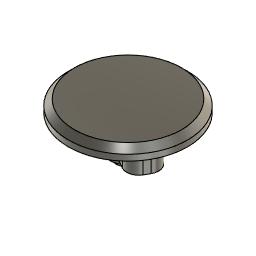
Scale_Hub_Long v2 (Autodesk Fusion 360 archive; units mm, degrees)
design "scaleHUB"
Autodesk Fusion 360 part; units mm, degrees
sketch "Sketch1" plane through (0, 0, 0) normal (0, 0, 1) x (1, 0, 0)
  line L0 (-2, 1.8875) -> (-2, -1.8875)
  line L1 (2, -1.8875) -> (2, 1.8875)
  line L2 (1.0213, 2.5533) -> (-1.0213, -2.5533) construction
  line L3 (-1.0213, 2.5533) -> (1.0213, -2.5533) construction
  arc A0 (2, 1.8875) -> (-2, 1.8875) centre (0, 0) ccw
  arc A1 (-2, -1.8875) -> (2, -1.8875) centre (0, 0) ccw
  circle A2 centre (0, 0) radius 6
  dimension "d1" = 5.5
  dimension "d4" = 12
  constraint coincident A0.centre A1.centre
  constraint parallel L0 L1
  constraint coincident L2 A0.centre
  constraint coincident L3 A0.centre
  constraint coincident L2.start A0
  constraint coincident L3.start A0
  constraint coincident L0.end A0
  constraint coincident L2.end A0
  constraint coincident L3.end A0
  constraint concentric A0 A1
  constraint concentric A0 A2
  measures "d1" diameter of A0
  measures "d4" diameter of A2
extrude "Extrude1" add sketch "Sketch1" along normal blind 7
chamfer "Chamfer1" distance 2 angle 45 1 edges at (-5.594, -2.1697, 0)
sketch "Sketch2" plane through (0, 0, 7) normal (0, 0, 1) x (-1, 0, 0)
  arc A0 (2, 1.8875) -> (-2, 1.8875) centre (0, 0) ccw
  line L0 (2, 1.8875) -> (2, -1.8875)
  arc A1 (-2, -1.8875) -> (2, -1.8875) centre (0, 0) ccw
  line L1 (-2, -1.8875) -> (-2, 1.8875)
  circle A2 centre (0, 0) radius 6
  circle A3 centre (0, 0) radius 7.5
  dimension "d8" = 15
  constraint coincident A0.centre A1.centre
  measures "d8" diameter of A3
extrude "Extrude2" add sketch "Sketch2" along normal blind 6 contours A2 | A3
sketch "Sketch3" plane through (0, 0, 13) normal (0, 0, 1) x (-1, 0, 0)
  arc A0 (2, 1.8875) -> (-2, 1.8875) centre (0, 0) ccw
  line L0 (2, 1.8875) -> (2, -1.8875)
  arc A1 (-2, -1.8875) -> (2, -1.8875) centre (0, 0) ccw
  line L1 (-2, -1.8875) -> (-2, 1.8875)
  circle A2 centre (0, 0) radius 7.5
  line L2 (0, -7.5) -> (0, -17.5) construction
  line L3 (0, -17.5) -> (5, -17.5) construction
  line L4 (5, -17.5) -> (-5, -17.5) construction
  line L5 (-5, -17.5) -> (-5, -5.5902) construction
  line L6 (5, -17.5) -> (5, -5.5902) construction
  line L7 (5, -5.5902) -> (5, -17.5)
  line L8 (-5, -17.5) -> (-5, -5.5902)
  line L9 (-5, -17.5) -> (5, -17.5)
  line L10 (17.6554, 4.4199) -> (7.3412, -1.535)
  line L11 (17.6554, 4.4199) -> (12.6554, 13.0801)
  line L12 (12.6554, 13.0801) -> (2.3412, 7.1252) construction
  line L13 (-12.6554, 13.0801) -> (-2.3412, 7.1252)
  line L14 (-12.6554, 13.0801) -> (-17.6554, 4.4199)
  line L15 (-17.6554, 4.4199) -> (-7.3412, -1.535) construction
  line L16 (-7.3412, -1.535) -> (-17.6554, 4.4199)
  line L17 (2.3412, 7.1252) -> (12.6554, 13.0801)
  dimension "d11" = 10
  dimension "d12" = 5
  dimension "d18" = 360
  constraint coincident A2 L2.start
  constraint vertical L2
  constraint perpendicular L2 L3
  constraint perpendicular L2 L4
  constraint coincident A2 L5.end
  constraint perpendicular L4 L5
  constraint coincident A2 L6.end
  constraint perpendicular L4 L6
  measures "d11" distance of L2.start L2.end
  measures "d12" distance of L2.end L3.end
extrude "Extrude3" add sketch "Sketch3" against normal blind 6 contours A2 L7 L8 L9
fillet "Fillet1" radius 5 2 edges at (5, 17.5, 10) (-5, 17.5, 10)
extrude "Extrude4" add sketch "Sketch3" against normal blind 6 contours A2 L10 L11 L17 | A2 L13 L14 L16 | A2 L7 L8 L9
fillet "Fillet2" radius 4 6 edges at (-5, 17.5, 10) (5, 17.5, 10) (17.6554, -4.4199, 10) (12.6554, -13.0801, 10) (-12.6554, -13.0801, 10) (-17.6554, -4.4199, 10)
sketch "Sketch4" plane through (0, 0, 13) normal (0, 0, 1) x (-1, 0, 0)
  arc A0 (14.1913, 2.4199) -> (15.6554, 7.884) centre (12.1913, 5.884) ccw
  line L0 (15.6554, 7.884) -> (14.6554, 9.616)
  arc A1 (14.6554, 9.616) -> (9.1913, 11.0801) centre (11.1913, 7.616) ccw
  line L1 (9.1913, 11.0801) -> (2.3412, 7.1252)
  arc A2 (2.3412, 7.1252) -> (-2.3412, 7.1252) centre (0, 0) ccw
  line L2 (-2.3412, 7.1252) -> (-9.1913, 11.0801)
  arc A3 (-9.1913, 11.0801) -> (-14.6554, 9.616) centre (-11.1913, 7.616) ccw
  line L3 (-14.6554, 9.616) -> (-15.6554, 7.884)
  arc A4 (-15.6554, 7.884) -> (-14.1913, 2.4199) centre (-12.1913, 5.884) ccw
  line L4 (-14.1913, 2.4199) -> (-7.3412, -1.535)
  arc A5 (-7.3412, -1.535) -> (-5, -5.5902) centre (0, 0) ccw
  line L5 (-5, -5.5902) -> (-5, -13.5)
  arc A6 (-5, -13.5) -> (-1, -17.5) centre (-1, -13.5) ccw
  line L6 (-1, -17.5) -> (1, -17.5)
  arc A7 (1, -17.5) -> (5, -13.5) centre (1, -13.5) ccw
  line L7 (5, -13.5) -> (5, -5.5902)
  arc A8 (5, -5.5902) -> (7.3412, -1.535) centre (0, 0) ccw
  line L8 (7.3412, -1.535) -> (14.1913, 2.4199)
  arc A9 (2, 1.8875) -> (-2, 1.8875) centre (0, 0) ccw
  line L9 (2, 1.8875) -> (2, -1.8875)
  arc A10 (-2, -1.8875) -> (2, -1.8875) centre (0, 0) ccw
  line L10 (-2, -1.8875) -> (-2, 1.8875)
  circle A11 centre (0, 0) radius 20
  dimension "d23" = 40
  constraint concentric A2 A11
  measures "d23" diameter of A11
extrude "Extrude5" add sketch "Sketch4" along normal blind 4 contours A0 L0 A1 L1 A2 L2 A3 L3 A4 L4 A5 L5 A6 L6 A7 L7 A8 L8 | A9 L9 A10 L10 | A11
chamfer "Chamfer2" distance 2 angle 45 1 edges at (18.6465, 7.2323, 17)
sketch "Sketch5" plane through (0, 0, 7) normal (0, 0, -1) x (1, 0, 0)
  arc A0 (-15.6554, 7.884) -> (-14.1913, 2.4199) centre (-12.1913, 5.884) ccw
  line L0 (-14.1913, 2.4199) -> (-7.3412, -1.535)
  arc A1 (-7.3412, -1.535) -> (-5, -5.5902) centre (0, 0) ccw
  line L1 (-5, -5.5902) -> (-5, -13.5)
  arc A2 (-5, -13.5) -> (-1, -17.5) centre (-1, -13.5) ccw
  line L2 (-1, -17.5) -> (1, -17.5)
  arc A3 (1, -17.5) -> (5, -13.5) centre (1, -13.5) ccw
  line L3 (5, -13.5) -> (5, -5.5902)
  arc A4 (5, -5.5902) -> (7.3412, -1.535) centre (0, 0) ccw
  line L4 (7.3412, -1.535) -> (14.1913, 2.4199)
  arc A5 (14.1913, 2.4199) -> (15.6554, 7.884) centre (12.1913, 5.884) ccw
  line L5 (15.6554, 7.884) -> (14.6554, 9.616)
  arc A6 (14.6554, 9.616) -> (9.1913, 11.0801) centre (11.1913, 7.616) ccw
  line L6 (9.1913, 11.0801) -> (2.3412, 7.1252)
  arc A7 (2.3412, 7.1252) -> (-2.3412, 7.1252) centre (0, 0) ccw
  line L7 (-2.3412, 7.1252) -> (-9.1913, 11.0801)
  arc A8 (-9.1913, 11.0801) -> (-14.6554, 9.616) centre (-11.1913, 7.616) ccw
  line L8 (-14.6554, 9.616) -> (-15.6554, 7.884)
  circle A9 centre (0, 0) radius 6
